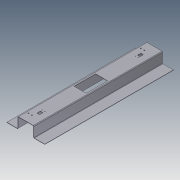
# Autodesk Inventor part: GE-12021
Saved by Autodesk Inventor 2012 (Build 160160000, 160)
## iProperties
Created: 2011-06-06
Part Number: GE-12021
Document SubType Name: Modeling
Designer: dfoster
Density: 7.85 g/cm^3
Material: Steel
Mass: 15023.8 g
Surface Area: 8423.68 cm^2
Volume: 1913.86 cm^3
Description: Bridge Base
Title: Bridge Base
Author: dfoster
Autodesk Inventor part; units mm, degrees
ref_plane "YZ Plane" through (0, 0, 0) normal (1, 0, 0) x (0, 1, 0)
ref_plane "XZ Plane" through (0, 0, 0) normal (0, 1, 0) x (-1, 0, 0)
sketch "Sketch1" plane through (0, 0, 0) normal (0, 0, 1) x (1, 0, 0)
  line L0 (0, 6.2128) -> (0, 95.3872)
  line L1 (6.2128, 101.6) -> (146.1872, 101.6)
  line L2 (152.4, 95.3872) -> (152.4, 6.2128)
  line L3 (149.3622, 6.2128) -> (149.3622, 95.3872)
  line L4 (146.1872, 98.5622) -> (6.2128, 98.5622)
  line L5 (3.0378, 95.3872) -> (3.0378, 6.2128)
  arc A0 (6.2128, 98.5622) -> (3.0378, 95.3872) centre (6.2128, 95.3872) ccw
  arc A1 (149.3622, 95.3872) -> (146.1872, 98.5622) centre (146.1872, 95.3872) ccw
  arc A2 (6.2128, 101.6) -> (0, 95.3872) centre (6.2128, 95.3872) ccw
  arc A3 (152.4, 95.3872) -> (146.1872, 101.6) centre (146.1872, 95.3872) ccw
  line L6 (-101.6, 0) -> (-3.175, 0)
  line L7 (-3.175, 3.0378) -> (-101.6, 3.0378)
  line L8 (-101.6, 3.0378) -> (-101.6, 0)
  line L9 (254, 0) -> (155.575, 0)
  line L10 (155.575, 3.0378) -> (254, 3.0378)
  line L11 (254, 3.0378) -> (254, 0)
  arc A4 (-3.175, 3.0378) -> (0, 6.2128) centre (-3.175, 6.2128) ccw
  arc A5 (152.4, 6.2128) -> (155.575, 3.0378) centre (155.575, 6.2128) ccw
  arc A6 (-3.175, 0) -> (3.0378, 6.2128) centre (-3.175, 6.2128) ccw
  arc A7 (149.3622, 6.2128) -> (155.575, 0) centre (155.575, 6.2128) ccw
  point P0 (0, 0)
  point P1 (0, 101.6)
  point P2 (152.4, 101.6)
  point P3 (152.4, 3.0378)
  point P4 (149.3622, 0)
  dimension "d0" = 101.6
  dimension "d1" = 3.0378
  dimension "d2" = 3.0378
  dimension "d3" = 152.4
  dimension "d4" = 3.175
  dimension "d5" = 6.2128
  dimension "d31" = 3.0378
  dimension "d32" = 3.0378
  dimension "d33" = 3.175
  dimension "d34" = 6.2128
  dimension "d35" = 101.6
  constraints: 24 end point, 16 point on circle, 16 tangent, 10 point on line, 8 centre point, 6 parallel, 4 equal radius, 3 vertical, 2 equal length, 2 horizontal, 1 collinear, 1 perpendicular
  measures "d0" distance of point (0, 0) point (0, 101.6)
  measures "d1" distance between parallel lines of L5 L0
  measures "d2" distance between parallel lines of L4 L1
  measures "d3" distance of point (0, 101.6) point (152.4, 101.6)
  measures "d4" radius of A0
  measures "d5" radius of A2
  measures "d31" distance between parallel lines of L6 L7
  measures "d32" distance between parallel lines of L2 L3
  measures "d33" radius of A4
  measures "d34" radius of A6
  measures "d35" distance between parallel lines of L8 L0
extrude "Extrusion1" add sketch "Sketch1" along normal blind 1206.5
hole "Hole1" at (25.4, 101.6, 1130.3) direction (0, -1, 0) diameter 9.906 end through all
pattern_linear "Rectangular Pattern1" count 2 spacing 31.75 along (1, 0, 0) of "Hole1"
pattern_linear "Rectangular Pattern2" count 2 spacing 1054.1 along (0, 0, -1) of "Hole1", "Rectangular Pattern1"
sketch "Sketch3" plane through (6.2128, 101.6, 0) normal (0, 1, 0) x (1, 0, 0)
  line L0 (0, -1206.5) -> (139.9743, -1206.5) projected
  line L1 (19.1872, -698.5) -> (120.7872, -698.5)
  line L2 (127.1372, -692.15) -> (127.1372, -501.65)
  line L3 (120.7872, -495.3) -> (19.1872, -495.3)
  line L4 (12.8372, -501.65) -> (12.8372, -692.15)
  arc A0 (12.8372, -692.15) -> (19.1872, -698.5) centre (19.1872, -692.15) ccw
  arc A1 (19.1872, -495.3) -> (12.8372, -501.65) centre (19.1872, -501.65) ccw
  arc A2 (127.1372, -501.65) -> (120.7872, -495.3) centre (120.7872, -501.65) ccw
  arc A3 (120.7872, -698.5) -> (127.1372, -692.15) centre (120.7872, -692.15) ccw
  line L5 (146.1872, 0) -> (146.1872, -1206.5) projected
  point P0 (-6.2128, 0)
  dimension "d36" = 6.35
  dimension "d37" = 203.2
  dimension "d38" = 114.3
  dimension "d39" = 19.05
  dimension "d40" = 508
  constraints: 8 end point, 8 point on circle, 8 tangent, 4 centre point, 3 equal radius, 2 parallel, 1 horizontal, 1 perpendicular
  measures "d36" radius of A0
  measures "d37" distance between parallel lines of L3 L1
  measures "d38" distance between parallel lines of L2 L4
  measures "d39" distance between parallel lines of L2 L5
  measures "d40" distance between parallel lines of L1 L0
extrude "Extrusion2" cut sketch "Sketch3" against normal blind 25.4
sketch "Sketch4" plane through (6.2128, 101.6, 0) normal (0, 1, 0) x (1, 0, 0)
  line L0 (0, -1206.5) -> (139.9743, -1206.5) projected
  line L1 (139.9743, 0) -> (139.9743, -1206.5) projected
  line L2 (0, 0) -> (0, -1206.5) projected
  line L3 (63.6372, -1092.2) -> (76.3372, -1092.2)
  line L4 (82.6872, -1085.85) -> (82.6872, -1063.625)
  line L5 (76.3372, -1057.275) -> (63.6372, -1057.275)
  line L6 (57.2872, -1063.625) -> (57.2872, -1085.85)
  arc A0 (57.2872, -1085.85) -> (63.6372, -1092.2) centre (63.6372, -1085.85) ccw
  arc A1 (76.3372, -1092.2) -> (82.6872, -1085.85) centre (76.3372, -1085.85) ccw
  arc A2 (82.6872, -1063.625) -> (76.3372, -1057.275) centre (76.3372, -1063.625) ccw
  arc A3 (63.6372, -1057.275) -> (57.2872, -1063.625) centre (63.6372, -1063.625) ccw
  point P0 (-6.2128, 0)
  point P1 (57.2872, -1092.2)
  point P2 (82.6872, -1057.275)
  point P3 (57.2872, -1057.275)
  dimension "d43" = 114.3
  dimension "d44" = 57.2872
  dimension "d45" = 25.4
  dimension "d46" = 139.9743
  dimension "d47" = 34.925
  dimension "d48" = 6.35
  constraints: 8 end point, 8 point on circle, 8 tangent, 6 point on line, 4 centre point, 3 equal radius, 2 parallel, 1 horizontal, 1 perpendicular
  measures "d43" distance between parallel lines of L3 L0
  measures "d44" distance between parallel lines of L4 L1
  measures "d45" distance of point (82.687, -1057.275) point (57.287, -1057.275)
  measures "d46" distance between parallel lines of L2 L1
  measures "d47" distance of point (57.287, -1057.275) point (57.287, -1092.2)
  measures "d48" radius of A0
extrude "Extrusion3" cut sketch "Sketch4" against normal blind 25.4
hole "Hole2" at (88.9, 101.6, 1041.4) direction (0, -1, 0) diameter 4.826 depth 25.4 tip angle 118
pattern_linear "Rectangular Pattern3" count 2 spacing 25.4 along (-1, 0, 0) of "Hole2"
ref_plane "Work Plane1" through (0, 0, 603.25) normal (0, 0, -1) x (-1, 0, 0)
mirror "Mirror1" about plane through (0, 0, 603.25) normal (0, 0, -1) of "Extrusion3", "Hole2", "Rectangular Pattern3"
equation "\"d2\" = d1"
equation "\"d5\" = d4 + d1"
equation "\"d31\" = d1"
equation "\"d32\" = d1"
equation "\"d33\" = d4"
equation "\"d34\" = d5"
equation "\"d44\" = -0.5 * d45 + 0.5 * d46"
body "Solid1"
